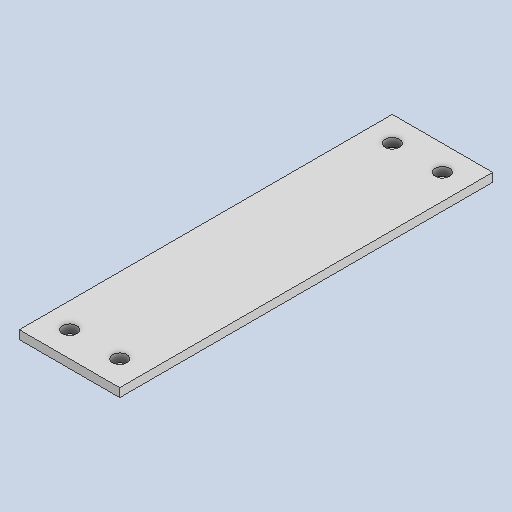
# Autodesk Inventor part: cap
Saved by Autodesk Inventor 2025 (Build 290162000, 162)
## iProperties
Created: 2025-08-20
Part Number: cap
Material: Generic
Document SubType Name: Modeling
Designer: Pravoslav
Density: 1 g/cm^3
Appearance: Default
Author: Pravoslav
Autodesk Inventor part; units mm, degrees
ref_plane "YZ Plane" through (0, 0, 0) normal (1, 0, 0) x (0, 1, 0)
ref_plane "XZ Plane" through (0, 0, 0) normal (0, 1, 0) x (-1, 0, 0)
ref_plane "XY Plane" through (0, 0, 0) normal (0, 0, 1) x (1, 0, 0)
sketch "Sketch1" plane through (0, 0, 0) normal (0, 1, 0) x (-1, 0, 0)
  line L0 (17.5, 65) -> (-17.5, 65)
  line L1 (-17.5, 65) -> (-17.5, -65)
  line L2 (-17.5, -65) -> (17.5, -65)
  line L3 (17.5, -65) -> (17.5, 65)
  line L4 (17.5, 65) -> (-17.5, -65) construction
  line L5 (-17.5, 65) -> (17.5, -65) construction
  line L6 (-17.5, 65) -> (0, 65)
  line L7 (0, 65) -> (0, 47.5)
  line L8 (0, 47.5) -> (-17.5, 47.5)
  line L9 (-17.5, 47.5) -> (-17.5, 65)
  line L10 (17.5, 65) -> (0, 65)
  line L11 (0, 65) -> (0, 47.5)
  line L12 (0, 47.5) -> (17.5, 47.5)
  line L13 (17.5, 47.5) -> (17.5, 65)
  line L14 (17.5, -65) -> (0, -65)
  line L15 (0, -65) -> (0, -47.5)
  line L16 (0, -47.5) -> (17.5, -47.5)
  line L17 (17.5, -47.5) -> (17.5, -65)
  line L18 (0, -47.5) -> (-17.5, -47.5)
  line L19 (-17.5, -47.5) -> (-17.5, -65)
  line L20 (-17.5, -65) -> (0, -65)
  line L21 (0, -65) -> (0, -47.5)
  circle A0 centre (8.75, 56.25) radius 2.5
  circle A1 centre (-8.75, 56.25) radius 2.5
  circle A2 centre (8.75, -56.25) radius 2.5
  circle A3 centre (-8.75, -56.25) radius 2.5
  point P0 (0, 0)
  dimension "d0" = 35
  dimension "d1" = 130
  dimension "d2" = 17.5
  dimension "d3" = 17.5
  dimension "d4" = 17.5
  dimension "d5" = 17.5
  dimension "d6" = 5
  dimension "d7" = 5
  dimension "d8" = 5
  dimension "d9" = 5
  dimension "d10" = 17.5
  dimension "d11" = 17.5
  dimension "d12" = 8.75
  dimension "d13" = 8.75
  dimension "d14" = 8.75
  dimension "d15" = 8.75
  dimension "d16" = 8.75
  dimension "d17" = 8.75
  constraints: 44 end point, 10 parallel, 5 horizontal, 5 perpendicular, 4 centre point, 2 midpoint
  measures "d0" distance of L2.end L1.end
  measures "d1" distance of L1.end L0.end
  measures "d2" distance of L7.end L8.end
  measures "d3" distance of L6.end L7.end
  measures "d4" distance of L15.end L16.end
  measures "d5" distance of L14.end L15.end
  measures "d6" diameter of A0
  measures "d7" diameter of A1
  measures "d8" diameter of A2
  measures "d9" diameter of A3
  measures "d10" distance of A2.centre A3.centre
  measures "d11" distance of A0.centre A1.centre
  measures "d12" distance from line of L13 A0.centre
  measures "d13" distance from line of L3 A2.centre
  measures "d14" distance from line of L2 A2.centre
  measures "d15" distance from line of L20 A3.centre
  measures "d16" distance from line of L0 A1.centre
  measures "d17" distance from line of L10 A0.centre
extrude "Extrusion1" add sketch "Sketch1" along normal blind 3
body "Solid1"
